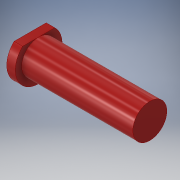
# Autodesk Inventor part: Idle pulley pin
Saved by Autodesk Inventor 2019.4 (Build 234330000, 330)
## iProperties
Created: 2020-02-23
Part Number: Idle pulley pin
Material: ABS Plastic
Document SubType Name: Modeling
Designer: admin
Density: 1.06 g/cm^3
Appearance: Red
Author: admin
Autodesk Inventor part; units mm, degrees
ref_plane "YZ Plane" through (0, 0, 0) normal (1, 0, 0) x (0, 1, 0)
ref_plane "XZ Plane" through (0, 0, 0) normal (0, 1, 0) x (-1, 0, 0)
ref_plane "XY Plane" through (0, 0, 0) normal (0, 0, 1) x (1, 0, 0)
sketch "Sketch1" plane through (0, 0, 0) normal (0, 0, 1) x (1, 0, 0)
  line L0 (0, 0) -> (0, 5.5)
  line L1 (0, 5.5) -> (2, 5.5)
  line L2 (2, 5.5) -> (2, 4)
  line L3 (2, 4) -> (7.1, 4)
  line L4 (7.1, 4) -> (7.1, 4)
  line L5 (7.1, 4) -> (8.2, 4)
  line L6 (8.2, 4) -> (8.2, 4)
  line L7 (8.2, 4) -> (9.1, 4)
  line L8 (9.1, 4) -> (9.1, 4)
  line L9 (9.1, 4) -> (10.1, 4)
  line L10 (10.1, 4) -> (10.1, 4)
  line L11 (10.1, 4) -> (26.1, 4)
  line L12 (26.1, 4) -> (26.1, 4)
  line L13 (26.1, 4) -> (27.1, 4)
  line L14 (27.1, 4) -> (27.1, 4)
  line L15 (27.1, 4) -> (28.1, 4)
  line L16 (28.1, 4) -> (28.1, 0)
  line L17 (28.1, 0) -> (0, 0)
  dimension "d0" = 2
  dimension "d1" = 4
  dimension "d2" = 1.5
  dimension "d3" = 1.1
  dimension "d4" = 0
  dimension "d5" = 1
  dimension "d6" = 1
  dimension "d7" = 1
  dimension "d8" = 16
  dimension "d9" = 5.1
  dimension "d10" = 3
  constraints: 36 end point, 12 perpendicular, 9 point on line, 1 parallel, 1 vertical
  measures "d0" distance of L0.end L1.end
  measures "d1" distance between parallel lines of L17 L3
  measures "d2" distance of L1.end L2.end
  measures "d3" distance of L4.end L5.end
  measures "d4" distance of L3.end L4.end
  measures "d5" distance of L12.end L13.end
  measures "d6" distance of L8.end L9.end
  measures "d7" distance of L14.end L15.end
  measures "d8" distance between parallel lines of L12 L10
  measures "d9" distance of L2.end L3.end
  measures "d10" distance between parallel lines of L10 L4
revolve "Revolution1" add sketch "Sketch1" angle 360 about axis through (28.1, 0, 0) along (-1, 0, 0)
sketch "Sketch2" plane through (2, 0, 0) normal (1, 0, 0) x (0, 0, -1)
  circle A0 centre (0, 0) radius 5.5 projected
  line L0 (-3.7749, 4) -> (3.7749, 4)
  circle A1 centre (0, 0) radius 4 projected
  point P0 (0, 0)
  constraints: 2 end point, 2 point on circle, 1 horizontal, 1 tangent
extrude "Extrusion1" cut sketch "Sketch2" against normal through all contours L0 A0 picked at (2.2014, 4.2388)
body "Solid1"
